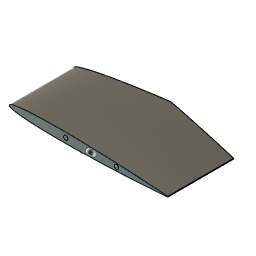
thrustVaneCFD-5deg (Autodesk Fusion 360 archive; units mm, degrees)
design "thrustVane1"
Autodesk Fusion 360 part; units mm, degrees
sketch "Sketch1" plane through (0, 0, 0) normal (0, 1, 0) x (1, 0, 0) in component "thrust vane"
ref_plane "WorkPlane1" through (0, 0.0001, 0) normal (0, 1, 0) x (0, 0, 1) in component "thrust vane"
sketch "NACA-M1_AIRFOIL_1.0" plane through (0, 0.0001, 0) normal (0, 1, 0) x (1, 0, 0)
  spline S0 degree 5 poles (60, -0.12) (59.8589, -0.1308) (59.5796, -0.1521) (59.1697, -0.1831) (58.6412, -0.2228) (58.0091, -0.2694) (57.4016, -0.3135) (56.8107, -0.3556) (56.223, -0.3966) (55.6192, -0.438) (54.9789, -0.4812) (54.2842, -0.5274) (53.5227, -0.5775) (52.6924, -0.6315) (51.8008, -0.689) (50.862, -0.7487) (49.8935, -0.8093) (48.9138, -0.8695) (47.9397, -0.928) (46.9829, -0.9838) (46.0483, -1.0368) (45.1348, -1.087) (44.2379, -1.1347) (43.3504, -1.1806) (42.4647, -1.2253) (41.5741, -1.2691) (40.6749, -1.3124) (39.7665, -1.3551) (38.8505, -1.3971) (37.9299, -1.438) (37.0084, -1.4774) (36.0891, -1.515) (35.1741, -1.5504) (34.2632, -1.5835) (33.355, -1.6143) (32.4469, -1.643) (31.5363, -1.6697) (30.6212, -1.6945) (29.7007, -1.7178) (28.7759, -1.7395) (27.8503, -1.7599) (26.928, -1.779) (26.0134, -1.7967) (25.1097, -1.8128) (24.218, -1.8272) (23.3365, -1.8396) (22.459, -1.8496) (21.5762, -1.8565) (20.6784, -1.8601) (19.7572, -1.8599) (18.8077, -1.8556) (17.8307, -1.8472) (16.8347, -1.8349) (15.8377, -1.8193) (14.862, -1.801) (13.9309, -1.7808) (13.064, -1.7593) (12.2739, -1.7372) (11.5618, -1.7144) (10.9125, -1.6906) (10.2979, -1.6652) (9.6875, -1.6371) (9.0562, -1.6055) (8.3935, -1.5699) (7.7127, -1.53) (7.0417, -1.4864) (6.4124, -1.4399) (5.8505, -1.3922) (5.3642, -1.3455) (4.9377, -1.3024) (4.5423, -1.2637) (4.1446, -1.2265) (3.7153, -1.1816) (3.2393, -1.1198) (2.7231, -1.0373) (2.2109, -0.9452) (1.7654, -0.8632) (1.4268, -0.8036) (1.1662, -0.7548) (0.8728, -0.6727) (0.4749, -0.516) (0.0866, -0.2813) (-0.0826, 0) (0.0866, 0.2813) (0.4749, 0.516) (0.8728, 0.6727) (1.1662, 0.7548) (1.4268, 0.8036) (1.7654, 0.8632) (2.2109, 0.9452) (2.7231, 1.0373) (3.2393, 1.1198) (3.7153, 1.1816) (4.1446, 1.2265) (4.5423, 1.2637) (4.9377, 1.3024) (5.3642, 1.3455) (5.8505, 1.3922) (6.4124, 1.4399) (7.0417, 1.4864) (7.7127, 1.53) (8.3935, 1.5699) (9.0562, 1.6055) (9.6875, 1.6371) (10.2979, 1.6652) (10.9125, 1.6906) (11.5618, 1.7144) (12.2739, 1.7372) (13.064, 1.7593) (13.9309, 1.7808) (14.862, 1.801) (15.8377, 1.8193) (16.8347, 1.8349) (17.8307, 1.8472) (18.8077, 1.8556) (19.7572, 1.8599) (20.6784, 1.8601) (21.5762, 1.8565) (22.459, 1.8496) (23.3365, 1.8396) (24.218, 1.8272) (25.1097, 1.8128) (26.0134, 1.7967) (26.928, 1.779) (27.8503, 1.7599) (28.7759, 1.7395) (29.7007, 1.7178) (30.6212, 1.6945) (31.5363, 1.6697) (32.4469, 1.643) (33.355, 1.6143) (34.2632, 1.5835) (35.1741, 1.5504) (36.0891, 1.515) (37.0084, 1.4774) (37.9299, 1.438) (38.8505, 1.3971) (39.7665, 1.3551) (40.6749, 1.3124) (41.5741, 1.2691) (42.4647, 1.2253) (43.3504, 1.1806) (44.2379, 1.1347) (45.1348, 1.087) (46.0483, 1.0368) (46.9829, 0.9838) (47.9397, 0.928) (48.9138, 0.8695) (49.8935, 0.8093) (50.862, 0.7487) (51.8008, 0.689) (52.6924, 0.6315) (53.5227, 0.5775) (54.2842, 0.5274) (54.9789, 0.4812) (55.6192, 0.438) (56.223, 0.3966) (56.8107, 0.3556) (57.4016, 0.3135) (58.0091, 0.2694) (58.6412, 0.2228) (59.1697, 0.1831) (59.5796, 0.1521) (59.8589, 0.1308) (60, 0.12) knots 0 0 0 0 0 0 0.00625 0.0125 0.01875 0.025 0.03125 0.0375 0.04375 0.05 0.05625 0.0625 0.06875 0.075 0.08125 0.0875 0.09375 0.1 0.10625 0.1125 0.11875 0.125 0.13125 0.1375 0.14375 0.15 0.15625 0.1625 0.16875 0.175 0.18125 0.1875 0.19375 0.2 0.20625 0.2125 0.21875 0.225 0.23125 0.2375 0.24375 0.25 0.25625 0.2625 0.26875 0.275 0.28125 0.2875 0.29375 0.3 0.30625 0.3125 0.31875 0.325 0.33125 0.3375 0.34375 0.35 0.35625 0.3625 0.36875 0.375 0.38125 0.3875 0.39375 0.4 0.40625 0.4125 0.41875 0.425 0.43125 0.4375 0.44375 0.45 0.45625 0.4625 0.46875 0.475 0.48125 0.4875 0.49375 0.5 0.50625 0.5125 0.51875 0.525 0.53125 0.5375 0.54375 0.55 0.55625 0.5625 0.56875 0.575 0.58125 0.5875 0.59375 0.6 0.60625 0.6125 0.61875 0.625 0.63125 0.6375 0.64375 0.65 0.65625 0.6625 0.66875 0.675 0.68125 0.6875 0.69375 0.7 0.70625 0.7125 0.71875 0.725 0.73125 0.7375 0.74375 0.75 0.75625 0.7625 0.76875 0.775 0.78125 0.7875 0.79375 0.8 0.80625 0.8125 0.81875 0.825 0.83125 0.8375 0.84375 0.85 0.85625 0.8625 0.86875 0.875 0.88125 0.8875 0.89375 0.9 0.90625 0.9125 0.91875 0.925 0.93125 0.9375 0.94375 0.95 0.95625 0.9625 0.96875 0.975 0.98125 0.9875 0.99375 1 1 1 1 1 1
  line L0 (60, -0.12) -> (60, 0.12)
  point P0 (57, -0.342)
  point P1 (54, -0.546)
  point P2 (48, -0.924)
  point P3 (42, -1.248)
  point P4 (36, -1.518)
  point P5 (30, -1.71)
  point P6 (24, -1.83)
  point P7 (18, -1.848)
  point P8 (12, -1.728)
  point P9 (9, -1.602)
  point P10 (6, -1.404)
  point P11 (4.5, -1.26)
  point P12 (3, -1.08)
  point P13 (1.5, -0.816)
  point P14 (0.75, -0.618)
  point P15 (0.75, 0.618)
  point P16 (1.5, 0.816)
  point P17 (3, 1.08)
  point P18 (4.5, 1.26)
  point P19 (6, 1.404)
  point P20 (9, 1.602)
  point P21 (12, 1.728)
  point P22 (18, 1.848)
  point P23 (24, 1.83)
  point P24 (30, 1.71)
  point P25 (36, 1.518)
  point P26 (42, 1.248)
  point P27 (48, 0.924)
  point P28 (54, 0.546)
  point P29 (57, 0.342)
  constraint vertical L0
extrude "Extrude1" add sketch "NACA-M1_AIRFOIL_1.0" along normal blind 30 in component "thrust vane"
scale "Scale1" factor 1.25 about (60, 0.0001, 0.12) bodies 1 in component "thrust vane"
sketch "Sketch4" plane through (0, 0.0001, 0) normal (0, -1, 0) x (1, 0, 0)
  line L0 (60, -0.18) -> (60, 0.12)
  spline S0 degree 5 poles (60, 0.12) (59.8236, 0.1335) (59.4745, 0.1601) (58.9622, 0.1989) (58.3015, 0.2484) (57.5114, 0.3068) (56.752, 0.3619) (56.0134, 0.4145) (55.2787, 0.4658) (54.524, 0.5175) (53.7237, 0.5715) (52.8553, 0.6292) (51.9034, 0.6918) (50.8655, 0.7594) (49.751, 0.8312) (48.5775, 0.9058) (47.3669, 0.9816) (46.1423, 1.0569) (44.9246, 1.13) (43.7286, 1.1998) (42.5603, 1.266) (41.4185, 1.3287) (40.2973, 1.3884) (39.188, 1.4458) (38.0809, 1.5016) (36.9677, 1.5564) (35.8436, 1.6105) (34.7081, 1.6639) (33.5631, 1.7164) (32.4124, 1.7675) (31.2605, 1.8168) (30.1113, 1.8637) (28.9676, 1.908) (27.829, 1.9494) (26.6937, 1.9879) (25.5586, 2.0238) (24.4203, 2.0571) (23.2765, 2.0882) (22.1258, 2.1172) (20.9699, 2.1444) (19.8129, 2.1699) (18.6601, 2.1937) (17.5168, 2.2158) (16.3871, 2.236) (15.2725, 2.2541) (14.1706, 2.2695) (13.0737, 2.2819) (11.9702, 2.2907) (10.848, 2.2952) (9.6965, 2.2949) (8.5096, 2.2895) (7.2883, 2.279) (6.0434, 2.2636) (4.7971, 2.2441) (3.5775, 2.2212) (2.4136, 2.1959) (1.3301, 2.1692) (0.3424, 2.1415) (-0.5477, 2.113) (-1.3594, 2.0833) (-2.1276, 2.0515) (-2.8907, 2.0164) (-3.6798, 1.9769) (-4.5082, 1.9324) (-5.3592, 1.8826) (-6.1978, 1.828) (-6.9845, 1.7699) (-7.6868, 1.7102) (-8.2948, 1.6518) (-8.8279, 1.598) (-9.3221, 1.5496) (-9.8192, 1.5031) (-10.3559, 1.447) (-10.9509, 1.3698) (-11.5961, 1.2667) (-12.2363, 1.1515) (-12.7932, 1.049) (-13.2165, 0.9745) (-13.5422, 0.9135) (-13.909, 0.8109) (-14.4063, 0.615) (-14.8917, 0.3216) (-15.1033, -0.03) (-14.8917, -0.3816) (-14.4063, -0.675) (-13.909, -0.8709) (-13.5422, -0.9735) (-13.2165, -1.0345) (-12.7932, -1.109) (-12.2363, -1.2115) (-11.5961, -1.3267) (-10.9509, -1.4298) (-10.3559, -1.507) (-9.8192, -1.5631) (-9.3221, -1.6096) (-8.8279, -1.658) (-8.2948, -1.7118) (-7.6868, -1.7702) (-6.9845, -1.8299) (-6.1978, -1.888) (-5.3592, -1.9426) (-4.5082, -1.9924) (-3.6798, -2.0369) (-2.8907, -2.0764) (-2.1276, -2.1115) (-1.3594, -2.1433) (-0.5477, -2.173) (0.3424, -2.2015) (1.3301, -2.2292) (2.4136, -2.2559) (3.5775, -2.2812) (4.7971, -2.3041) (6.0434, -2.3236) (7.2883, -2.339) (8.5096, -2.3495) (9.6965, -2.3549) (10.848, -2.3552) (11.9702, -2.3507) (13.0737, -2.3419) (14.1706, -2.3295) (15.2725, -2.3141) (16.3871, -2.296) (17.5168, -2.2758) (18.6601, -2.2537) (19.8129, -2.2299) (20.9699, -2.2044) (22.1258, -2.1772) (23.2765, -2.1482) (24.4203, -2.1171) (25.5586, -2.0838) (26.6937, -2.0479) (27.829, -2.0094) (28.9676, -1.968) (30.1113, -1.9237) (31.2605, -1.8768) (32.4124, -1.8275) (33.5631, -1.7764) (34.7081, -1.7239) (35.8436, -1.6705) (36.9677, -1.6164) (38.0809, -1.5616) (39.188, -1.5058) (40.2973, -1.4484) (41.4185, -1.3887) (42.5603, -1.326) (43.7286, -1.2598) (44.9246, -1.19) (46.1423, -1.1169) (47.3669, -1.0416) (48.5775, -0.9658) (49.751, -0.8912) (50.8655, -0.8194) (51.9034, -0.7518) (52.8553, -0.6892) (53.7237, -0.6315) (54.524, -0.5775) (55.2787, -0.5258) (56.0134, -0.4745) (56.752, -0.4219) (57.5114, -0.3668) (58.3015, -0.3084) (58.9622, -0.2589) (59.4745, -0.2201) (59.8236, -0.1935) (60, -0.18) knots 0 0 0 0 0 0 0.00625 0.0125 0.01875 0.025 0.03125 0.0375 0.04375 0.05 0.05625 0.0625 0.06875 0.075 0.08125 0.0875 0.09375 0.1 0.10625 0.1125 0.11875 0.125 0.13125 0.1375 0.14375 0.15 0.15625 0.1625 0.16875 0.175 0.18125 0.1875 0.19375 0.2 0.20625 0.2125 0.21875 0.225 0.23125 0.2375 0.24375 0.25 0.25625 0.2625 0.26875 0.275 0.28125 0.2875 0.29375 0.3 0.30625 0.3125 0.31875 0.325 0.33125 0.3375 0.34375 0.35 0.35625 0.3625 0.36875 0.375 0.38125 0.3875 0.39375 0.4 0.40625 0.4125 0.41875 0.425 0.43125 0.4375 0.44375 0.45 0.45625 0.4625 0.46875 0.475 0.48125 0.4875 0.49375 0.5 0.50625 0.5125 0.51875 0.525 0.53125 0.5375 0.54375 0.55 0.55625 0.5625 0.56875 0.575 0.58125 0.5875 0.59375 0.6 0.60625 0.6125 0.61875 0.625 0.63125 0.6375 0.64375 0.65 0.65625 0.6625 0.66875 0.675 0.68125 0.6875 0.69375 0.7 0.70625 0.7125 0.71875 0.725 0.73125 0.7375 0.74375 0.75 0.75625 0.7625 0.76875 0.775 0.78125 0.7875 0.79375 0.8 0.80625 0.8125 0.81875 0.825 0.83125 0.8375 0.84375 0.85 0.85625 0.8625 0.86875 0.875 0.88125 0.8875 0.89375 0.9 0.90625 0.9125 0.91875 0.925 0.93125 0.9375 0.94375 0.95 0.95625 0.9625 0.96875 0.975 0.98125 0.9875 0.99375 1 1 1 1 1 1
sketch "Sketch5" plane through (0, 0.0001, 0) normal (0, -1, 0) x (1, 0, 0)
  line L0 (-15, 0) -> (3.75, 0)
  line L1 (3.75, 0) -> (23.75, 0)
  line L2 (23.75, 0) -> (35.75, 0)
  line L3 (23.75, 0) -> (11.75, 0)
  circle A0 centre (11.75, 0) radius 1
  circle A1 centre (35.75, 0) radius 1
  circle A2 centre (23.75, 0) radius 1
  point P0 (23.75, 0)
  point P1 (23.75, 0)
  dimension "d19" = 18.75
  dimension "d20" = 20
  dimension "d21" = 12
  dimension "d22" = 12
  dimension "d23" = 2
  dimension "d24" = 2
  dimension "d25" = 2
  constraint horizontal L0
  constraint parallel L0 L1
  constraint coincident P1 P0
  constraint parallel L1 L2
  constraint parallel L1 L3
  constraint coincident L3.end A0.centre
  constraint coincident L2.end A1.centre
  measures "d19" distance of L0.start L0.end
  measures "d20" distance of L0.end P1
  measures "d21" distance of P1 L2.end
  measures "d22" distance of P1 L3.end
  measures "d23" diameter of A0
  measures "d24" diameter of A1
  measures "d25" diameter of A2
extrude "Extrude3" cut sketch "Sketch5" against normal blind 6 contours L1 L3 A0 | L1 L3 A0 | A1 in component "thrust vane"
sketch "Sketch6" plane through (0, 0.0001, 0) normal (0, -1, 0) x (1, 0, 0)
  line L0 (-15, 0) -> (3.75, 0)
  line L1 (3.75, 0) -> (23.75, 0)
  circle A0 centre (23.75, 0) radius 1
  dimension "d28" = 18.75
  dimension "d29" = 20
  dimension "d30" = 2
  constraint horizontal L0
  constraint parallel L0 L1
  constraint coincident L1.end A0.centre
  measures "d28" distance of L0.start L0.end
  measures "d29" distance of L0.end L1.end
  measures "d30" diameter of A0
extrude "Extrude4" cut sketch "Sketch6" against normal blind 1 in component "thrust vane"
sketch "Sketch7" plane through (0, 0, 0) normal (0, 0, 1) x (1, 0, 0)
  line L0 (60, 37.5) -> (60, 29.5)
  line L1 (60, 37.5) -> (22.5, 37.5)
  line L2 (60, 29.5) -> (22.5, 37.5)
  line L3 (22.5, 37.5) -> (-15.2023, 33.5)
  line L4 (22.5, 37.5) -> (-15, 37.5)
  line L5 (-15, 37.5) -> (-15.2023, 33.5)
  dimension "d33" = 8
  dimension "d34" = 37.5
  constraint vertical L0
  constraint perpendicular L0 L1
  constraint horizontal L4
  measures "d33" distance of L0.start L0.end
  measures "d34" distance of L0.start L1.end
sketch "Sketch9" plane through (0, 0, 0) normal (0, 0, 1) x (1, 0, 0)
sketch "Sketch10" plane through (0, 0.0001, 0) normal (0, -1, 0) x (1, 0, 0)
  line L0 (22.75, 0) -> (24.75, 0)
  constraint horizontal L0
sketch "Sketch11" plane through (0, 0, 0) normal (0, 1, 0) x (1, 0, 0)
sketch "Sketch12" plane through (0, 0.0001, 0) normal (0, -1, 0) x (1, 0, 0)
  line L0 (22.75, 0) -> (23.75, 0)
  point P0 (23.75, 0)
  dimension "d43" = 1
  constraint horizontal L0
  constraint coincident P0 L0.end
  measures "d43" distance of L0.start P0
sketch "Sketch13" plane through (0, 0, 0) normal (0, 0, 1) x (1, 0, 0)
  line L0 (23.75, 0) -> (23.75, 37.5)
  line L1 (23.75, 37.5) -> (-15.6462, 30.5534)
  line L2 (23.75, 37.5) -> (62.2681, 34.0267)
  line L3 (62.2681, 34.0267) -> (62.2681, 40)
  line L4 (62.2681, 40) -> (-16, 40)
  line L5 (-16, 40) -> (-15.6462, 30.5534)
  dimension "d44" = 80
  constraint vertical L0
  constraint parallel L0 L3
  constraint perpendicular L0 L4
  measures "d44" angle of L0 L1
extrude "Extrude8" cut sketch "Sketch13" along normal mid plane 8 in component "thrust vane"
sketch "Sketch14" plane through (0, 0, 0) normal (0, 0, 1) x (1, 0, 0)
  line L0 (23.75, 0) -> (23.75, 37.585)
  line L1 (23.75, 37.585) -> (61.3996, 30.9464)
  line L2 (61.3996, 30.9464) -> (61.3996, 37.585)
  line L3 (61.3996, 37.585) -> (23.75, 37.585)
  dimension "d47" = 80
  constraint vertical L0
  constraint parallel L0 L2
  constraint perpendicular L0 L3
  measures "d47" angle of L0 L1
extrude "Extrude9" cut sketch "Sketch14" along normal mid plane 14 in component "thrust vane"
extrude "Extrude5" [suppressed] in component "thrust vane"
sketch "Sketch8" plane through (0, 0, 0) normal (0, 0, 1) x (1, 0, 0)
  line L0 (60, 37.5) -> (60, 29.5)
  line L1 (60, 29.5) -> (23.9967, 37.5263)
  line L2 (23.9967, 37.5263) -> (60, 37.5)
  dimension "d37" = 8
  constraint vertical L0
  measures "d37" distance of L0.start L0.end
extrude "Extrude6" [suppressed] in component "thrust vane"
extrude "Extrude7" [suppressed] in component "thrust vane"
chamfer "Chamfer1" [suppressed] in component "thrust vane"
sketch "Sketch2" plane through (0, 0.0001, 0) normal (0, -1, 0) x (1, 0, 0)
  line L0 (60, -0.12) -> (60, 0.12)
  spline S0 degree 5 poles (60, 0.12) (59.8589, 0.1308) (59.5796, 0.1521) (59.1697, 0.1831) (58.6412, 0.2228) (58.0091, 0.2694) (57.4016, 0.3135) (56.8107, 0.3556) (56.223, 0.3966) (55.6192, 0.438) (54.9789, 0.4812) (54.2842, 0.5274) (53.5227, 0.5775) (52.6924, 0.6315) (51.8008, 0.689) (50.862, 0.7487) (49.8935, 0.8093) (48.9138, 0.8695) (47.9397, 0.928) (46.9829, 0.9838) (46.0483, 1.0368) (45.1348, 1.087) (44.2379, 1.1347) (43.3504, 1.1806) (42.4647, 1.2253) (41.5741, 1.2691) (40.6749, 1.3124) (39.7665, 1.3551) (38.8505, 1.3971) (37.9299, 1.438) (37.0084, 1.4774) (36.0891, 1.515) (35.1741, 1.5504) (34.2632, 1.5835) (33.355, 1.6143) (32.4469, 1.643) (31.5363, 1.6697) (30.6212, 1.6945) (29.7007, 1.7178) (28.7759, 1.7395) (27.8503, 1.7599) (26.928, 1.779) (26.0134, 1.7967) (25.1097, 1.8128) (24.218, 1.8272) (23.3365, 1.8396) (22.459, 1.8496) (21.5762, 1.8565) (20.6784, 1.8601) (19.7572, 1.8599) (18.8077, 1.8556) (17.8307, 1.8472) (16.8347, 1.8349) (15.8377, 1.8193) (14.862, 1.801) (13.9309, 1.7808) (13.064, 1.7593) (12.2739, 1.7372) (11.5618, 1.7144) (10.9125, 1.6906) (10.2979, 1.6652) (9.6875, 1.6371) (9.0562, 1.6055) (8.3935, 1.5699) (7.7127, 1.53) (7.0417, 1.4864) (6.4124, 1.4399) (5.8505, 1.3922) (5.3642, 1.3455) (4.9377, 1.3024) (4.5423, 1.2637) (4.1446, 1.2265) (3.7153, 1.1816) (3.2393, 1.1198) (2.7231, 1.0373) (2.2109, 0.9452) (1.7654, 0.8632) (1.4268, 0.8036) (1.1662, 0.7548) (0.8728, 0.6727) (0.4749, 0.516) (0.0866, 0.2813) (-0.0826, 0) (0.0866, -0.2813) (0.4749, -0.516) (0.8728, -0.6727) (1.1662, -0.7548) (1.4268, -0.8036) (1.7654, -0.8632) (2.2109, -0.9452) (2.7231, -1.0373) (3.2393, -1.1198) (3.7153, -1.1816) (4.1446, -1.2265) (4.5423, -1.2637) (4.9377, -1.3024) (5.3642, -1.3455) (5.8505, -1.3922) (6.4124, -1.4399) (7.0417, -1.4864) (7.7127, -1.53) (8.3935, -1.5699) (9.0562, -1.6055) (9.6875, -1.6371) (10.2979, -1.6652) (10.9125, -1.6906) (11.5618, -1.7144) (12.2739, -1.7372) (13.064, -1.7593) (13.9309, -1.7808) (14.862, -1.801) (15.8377, -1.8193) (16.8347, -1.8349) (17.8307, -1.8472) (18.8077, -1.8556) (19.7572, -1.8599) (20.6784, -1.8601) (21.5762, -1.8565) (22.459, -1.8496) (23.3365, -1.8396) (24.218, -1.8272) (25.1097, -1.8128) (26.0134, -1.7967) (26.928, -1.779) (27.8503, -1.7599) (28.7759, -1.7395) (29.7007, -1.7178) (30.6212, -1.6945) (31.5363, -1.6697) (32.4469, -1.643) (33.355, -1.6143) (34.2632, -1.5835) (35.1741, -1.5504) (36.0891, -1.515) (37.0084, -1.4774) (37.9299, -1.438) (38.8505, -1.3971) (39.7665, -1.3551) (40.6749, -1.3124) (41.5741, -1.2691) (42.4647, -1.2253) (43.3504, -1.1806) (44.2379, -1.1347) (45.1348, -1.087) (46.0483, -1.0368) (46.9829, -0.9838) (47.9397, -0.928) (48.9138, -0.8695) (49.8935, -0.8093) (50.862, -0.7487) (51.8008, -0.689) (52.6924, -0.6315) (53.5227, -0.5775) (54.2842, -0.5274) (54.9789, -0.4812) (55.6192, -0.438) (56.223, -0.3966) (56.8107, -0.3556) (57.4016, -0.3135) (58.0091, -0.2694) (58.6412, -0.2228) (59.1697, -0.1831) (59.5796, -0.1521) (59.8589, -0.1308) (60, -0.12) knots 0 0 0 0 0 0 0.00625 0.0125 0.01875 0.025 0.03125 0.0375 0.04375 0.05 0.05625 0.0625 0.06875 0.075 0.08125 0.0875 0.09375 0.1 0.10625 0.1125 0.11875 0.125 0.13125 0.1375 0.14375 0.15 0.15625 0.1625 0.16875 0.175 0.18125 0.1875 0.19375 0.2 0.20625 0.2125 0.21875 0.225 0.23125 0.2375 0.24375 0.25 0.25625 0.2625 0.26875 0.275 0.28125 0.2875 0.29375 0.3 0.30625 0.3125 0.31875 0.325 0.33125 0.3375 0.34375 0.35 0.35625 0.3625 0.36875 0.375 0.38125 0.3875 0.39375 0.4 0.40625 0.4125 0.41875 0.425 0.43125 0.4375 0.44375 0.45 0.45625 0.4625 0.46875 0.475 0.48125 0.4875 0.49375 0.5 0.50625 0.5125 0.51875 0.525 0.53125 0.5375 0.54375 0.55 0.55625 0.5625 0.56875 0.575 0.58125 0.5875 0.59375 0.6 0.60625 0.6125 0.61875 0.625 0.63125 0.6375 0.64375 0.65 0.65625 0.6625 0.66875 0.675 0.68125 0.6875 0.69375 0.7 0.70625 0.7125 0.71875 0.725 0.73125 0.7375 0.74375 0.75 0.75625 0.7625 0.76875 0.775 0.78125 0.7875 0.79375 0.8 0.80625 0.8125 0.81875 0.825 0.83125 0.8375 0.84375 0.85 0.85625 0.8625 0.86875 0.875 0.88125 0.8875 0.89375 0.9 0.90625 0.9125 0.91875 0.925 0.93125 0.9375 0.94375 0.95 0.95625 0.9625 0.96875 0.975 0.98125 0.9875 0.99375 1 1 1 1 1 1
  line L1 (0, 0) -> (15, 0)
  line L2 (15, 0) -> (35, 0)
  line L3 (35, 0) -> (21.4, 0)
  line L4 (35, 0) -> (48.6, 0)
  line L5 (21.4, 0) -> (23.1, 0)
  line L6 (48.6, 0) -> (46.9, 0)
  line L7 (23.1, 0) -> (28.1, 0)
  line L8 (46.9, 0) -> (41.9, 0)
  circle A0 centre (23.1, 0) radius 1
  circle A1 centre (28.1, 0) radius 1
  circle A2 centre (41.9, 0) radius 1
  point P0 (15, 0)
  point P1 (35, 0)
  point P2 (28.1, 0)
  point P3 (21.4, 0)
  point P4 (23.1, 0)
  point P5 (46.9, 0)
  point P6 (48.6, 0)
  dimension "d4" = 15
  dimension "d5" = 20
  dimension "d6" = 13.6
  dimension "d7" = 13.6
  dimension "d8" = 1.7
  dimension "d9" = 1.7
  dimension "d10" = 5
  dimension "d11" = 5
  dimension "d12" = 2
  dimension "d13" = 2
  dimension "d14" = 2
  constraint horizontal L1
  constraint coincident L1.start origin
  constraint coincident P0 L1.end
  constraint parallel L1 L2
  constraint parallel L2 L3
  constraint parallel L2 L4
  constraint parallel L3 L5
  constraint parallel L4 L6
  constraint parallel L2 L7
  constraint parallel L4 L8
  constraint coincident P1 L2.end
  constraint coincident P2 L7.end
  constraint coincident P3 L3.end
  constraint coincident P4 L5.end
  constraint coincident P5 L6.end
  constraint coincident P6 L4.end
  constraint coincident L8.end A2.centre
  measures "d4" distance of L1.start P0
  measures "d5" distance of P0 P1
  measures "d6" distance of P1 P3
  measures "d7" distance of P1 P6
  measures "d8" distance of P3 P4
  measures "d9" distance of P6 P5
  measures "d10" distance of P4 P2
  measures "d11" distance of P5 L8.end
  measures "d12" diameter of A0
  measures "d13" diameter of A1
  measures "d14" diameter of A2
extrude "Extrude2" [suppressed] in component "thrust vane"
sketch "Sketch3" plane through (0, 0.0001, 0) normal (0, -1, 0) x (1, 0, 0)
  circle A0 centre (23.1, 0) radius 1
  circle A1 centre (28.1, 0) radius 1
  circle A2 centre (41.9, 0) radius 1
  line L0 (60, -0.12) -> (60, 0.12)
  spline S0 degree 5 poles (60, 0.12) (59.8589, 0.1308) (59.5796, 0.1521) (59.1697, 0.1831) (58.6412, 0.2228) (58.0091, 0.2694) (57.4016, 0.3135) (56.8107, 0.3556) (56.223, 0.3966) (55.6192, 0.438) (54.9789, 0.4812) (54.2842, 0.5274) (53.5227, 0.5775) (52.6924, 0.6315) (51.8008, 0.689) (50.862, 0.7487) (49.8935, 0.8093) (48.9138, 0.8695) (47.9397, 0.928) (46.9829, 0.9838) (46.0483, 1.0368) (45.1348, 1.087) (44.2379, 1.1347) (43.3504, 1.1806) (42.4647, 1.2253) (41.5741, 1.2691) (40.6749, 1.3124) (39.7665, 1.3551) (38.8505, 1.3971) (37.9299, 1.438) (37.0084, 1.4774) (36.0891, 1.515) (35.1741, 1.5504) (34.2632, 1.5835) (33.355, 1.6143) (32.4469, 1.643) (31.5363, 1.6697) (30.6212, 1.6945) (29.7007, 1.7178) (28.7759, 1.7395) (27.8503, 1.7599) (26.928, 1.779) (26.0134, 1.7967) (25.1097, 1.8128) (24.218, 1.8272) (23.3365, 1.8396) (22.459, 1.8496) (21.5762, 1.8565) (20.6784, 1.8601) (19.7572, 1.8599) (18.8077, 1.8556) (17.8307, 1.8472) (16.8347, 1.8349) (15.8377, 1.8193) (14.862, 1.801) (13.9309, 1.7808) (13.064, 1.7593) (12.2739, 1.7372) (11.5618, 1.7144) (10.9125, 1.6906) (10.2979, 1.6652) (9.6875, 1.6371) (9.0562, 1.6055) (8.3935, 1.5699) (7.7127, 1.53) (7.0417, 1.4864) (6.4124, 1.4399) (5.8505, 1.3922) (5.3642, 1.3455) (4.9377, 1.3024) (4.5423, 1.2637) (4.1446, 1.2265) (3.7153, 1.1816) (3.2393, 1.1198) (2.7231, 1.0373) (2.2109, 0.9452) (1.7654, 0.8632) (1.4268, 0.8036) (1.1662, 0.7548) (0.8728, 0.6727) (0.4749, 0.516) (0.0866, 0.2813) (-0.0826, 0) (0.0866, -0.2813) (0.4749, -0.516) (0.8728, -0.6727) (1.1662, -0.7548) (1.4268, -0.8036) (1.7654, -0.8632) (2.2109, -0.9452) (2.7231, -1.0373) (3.2393, -1.1198) (3.7153, -1.1816) (4.1446, -1.2265) (4.5423, -1.2637) (4.9377, -1.3024) (5.3642, -1.3455) (5.8505, -1.3922) (6.4124, -1.4399) (7.0417, -1.4864) (7.7127, -1.53) (8.3935, -1.5699) (9.0562, -1.6055) (9.6875, -1.6371) (10.2979, -1.6652) (10.9125, -1.6906) (11.5618, -1.7144) (12.2739, -1.7372) (13.064, -1.7593) (13.9309, -1.7808) (14.862, -1.801) (15.8377, -1.8193) (16.8347, -1.8349) (17.8307, -1.8472) (18.8077, -1.8556) (19.7572, -1.8599) (20.6784, -1.8601) (21.5762, -1.8565) (22.459, -1.8496) (23.3365, -1.8396) (24.218, -1.8272) (25.1097, -1.8128) (26.0134, -1.7967) (26.928, -1.779) (27.8503, -1.7599) (28.7759, -1.7395) (29.7007, -1.7178) (30.6212, -1.6945) (31.5363, -1.6697) (32.4469, -1.643) (33.355, -1.6143) (34.2632, -1.5835) (35.1741, -1.5504) (36.0891, -1.515) (37.0084, -1.4774) (37.9299, -1.438) (38.8505, -1.3971) (39.7665, -1.3551) (40.6749, -1.3124) (41.5741, -1.2691) (42.4647, -1.2253) (43.3504, -1.1806) (44.2379, -1.1347) (45.1348, -1.087) (46.0483, -1.0368) (46.9829, -0.9838) (47.9397, -0.928) (48.9138, -0.8695) (49.8935, -0.8093) (50.862, -0.7487) (51.8008, -0.689) (52.6924, -0.6315) (53.5227, -0.5775) (54.2842, -0.5274) (54.9789, -0.4812) (55.6192, -0.438) (56.223, -0.3966) (56.8107, -0.3556) (57.4016, -0.3135) (58.0091, -0.2694) (58.6412, -0.2228) (59.1697, -0.1831) (59.5796, -0.1521) (59.8589, -0.1308) (60, -0.12) knots 0 0 0 0 0 0 0.00625 0.0125 0.01875 0.025 0.03125 0.0375 0.04375 0.05 0.05625 0.0625 0.06875 0.075 0.08125 0.0875 0.09375 0.1 0.10625 0.1125 0.11875 0.125 0.13125 0.1375 0.14375 0.15 0.15625 0.1625 0.16875 0.175 0.18125 0.1875 0.19375 0.2 0.20625 0.2125 0.21875 0.225 0.23125 0.2375 0.24375 0.25 0.25625 0.2625 0.26875 0.275 0.28125 0.2875 0.29375 0.3 0.30625 0.3125 0.31875 0.325 0.33125 0.3375 0.34375 0.35 0.35625 0.3625 0.36875 0.375 0.38125 0.3875 0.39375 0.4 0.40625 0.4125 0.41875 0.425 0.43125 0.4375 0.44375 0.45 0.45625 0.4625 0.46875 0.475 0.48125 0.4875 0.49375 0.5 0.50625 0.5125 0.51875 0.525 0.53125 0.5375 0.54375 0.55 0.55625 0.5625 0.56875 0.575 0.58125 0.5875 0.59375 0.6 0.60625 0.6125 0.61875 0.625 0.63125 0.6375 0.64375 0.65 0.65625 0.6625 0.66875 0.675 0.68125 0.6875 0.69375 0.7 0.70625 0.7125 0.71875 0.725 0.73125 0.7375 0.74375 0.75 0.75625 0.7625 0.76875 0.775 0.78125 0.7875 0.79375 0.8 0.80625 0.8125 0.81875 0.825 0.83125 0.8375 0.84375 0.85 0.85625 0.8625 0.86875 0.875 0.88125 0.8875 0.89375 0.9 0.90625 0.9125 0.91875 0.925 0.93125 0.9375 0.94375 0.95 0.95625 0.9625 0.96875 0.975 0.98125 0.9875 0.99375 1 1 1 1 1 1
component "thrust vane" placed x (1, 0, 0) y (0, 1, 0) z (0, 0, 1) at (0, 0, 0)
equation "d4 = ( 60.000 * 0.25 ) * 1 mm"
equation "d19 = ( 75 / 4 ) * 1 mm"
equation "d28 = ( 75 / 4 ) * 1 mm"
equation "d34 = ( 75.000 / 2 ) * 1 mm"
equation "d44 = 90 deg - 10 deg"
